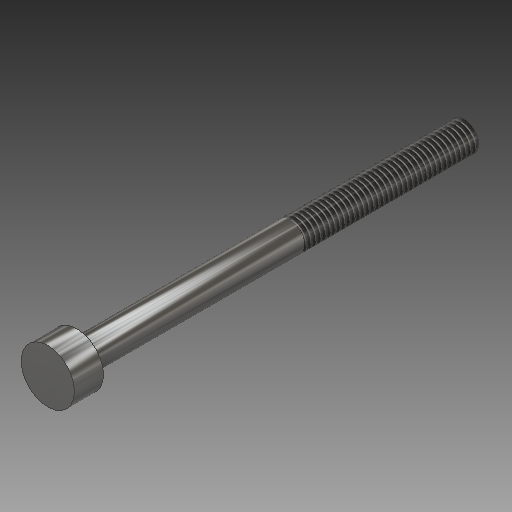
# Autodesk Inventor part: ネジキャップm3,40
Saved by Autodesk Inventor 2020 (Build 240168000, 168)
## iProperties
Created: 2018-12-30
Part Number: ネジキャップm3,40
Material: 鋼、高強度、低合金
Document SubType Name: Modeling
Designer: 雪村
Density: 7.85 g/cm^3
Appearance: 鋼 - つや出し
Mass: 2.77904 g
Surface Area: 4.76344 cm^2
Volume: 0.354018 cm^3
Author: 雪村
Autodesk Inventor part; units mm, degrees
ref_plane "YZ Plane" through (0, 0, 0) normal (1, 0, 0) x (0, 1, 0)
ref_plane "XZ Plane" through (0, 0, 0) normal (0, 1, 0) x (-1, 0, 0)
ref_plane "XY Plane" through (0, 0, 0) normal (0, 0, 1) x (1, 0, 0)
sketch "スケッチ1" plane through (0, 0, 0) normal (0, 0, 1) x (1, 0, 0)
  circle A0 centre (0, 0) radius 2.75
  dimension "d0" = 5.5
  constraints: 1 centre point, 1 coincident
  measures "d0" diameter of A0
extrude "押し出し1" add sketch "スケッチ1" along normal blind 3
sketch "スケッチ2" plane through (0, 0, 0) normal (0, 0, -1) x (-1, 0, 0)
  circle A0 centre (0, 0) radius 1.5
  dimension "d3" = 3
  constraints: 1 centre point, 1 coincident
  measures "d3" diameter of A0
extrude "押し出し2" add sketch "スケッチ2" along normal blind 40
thread "ねじ1" size "M3x0.5" class "6g" standard "ANSI Metric M Profile" length 18
